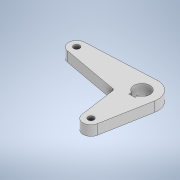
# Autodesk Inventor part: Part3
Saved by Autodesk Inventor 2021 (Build 250183000, 183)
## iProperties
Created: 2022-04-24
Part Number: Part3
Material: Generic
Document SubType Name: Modeling
Designer: hp
Density: 1 g/cm^3
Appearance: Default
Author: hp
Autodesk Inventor part; units mm, degrees
ref_plane "YZ Plane" through (0, 0, 0) normal (1, 0, 0) x (0, 1, 0)
ref_plane "XZ Plane" through (0, 0, 0) normal (0, 1, 0) x (-1, 0, 0)
ref_plane "XY Plane" through (0, 0, 0) normal (0, 0, 1) x (1, 0, 0)
sketch "Sketch1" plane through (0, 0, 0) normal (0, 1, 0) x (-1, 0, 0)
  arc A0 (32.9765, -145.5888) -> (49.4852, -164.4428) centre (48.7166, -148.4613) ccw
  arc A1 (119.1009, -161.0946) -> (120.1528, -145.2338) centre (118.7166, -153.1038) ccw
  arc A2 (57.63, -97.3385) -> (41.8392, -97.025) centre (49.7092, -98.4613) ccw
  line L0 (41.8392, -97.025) -> (32.9765, -145.5888)
  line L1 (49.4852, -164.4428) -> (119.1009, -161.0946)
  line L2 (120.1528, -145.2338) -> (64.3577, -135.0515)
  line L3 (57.63, -97.3385) -> (62.7366, -133.3646)
  circle A3 centre (49.7092, -98.4613) radius 3
  arc A4 (45.7166, -141.0451) -> (51.7166, -141.0451) centre (48.7166, -148.4613) ccw
  circle A5 centre (118.7166, -153.1038) radius 3
  line L4 (51.7166, -138.4613) -> (45.7166, -138.4613)
  line L5 (51.7166, -156.4613) -> (51.7166, -155.8775)
  line L6 (51.7166, -141.0451) -> (51.7166, -138.4613)
  line L7 (45.7166, -138.4613) -> (45.7166, -141.0451)
  arc A6 (62.7366, -133.3646) -> (64.3577, -135.0515) centre (64.7168, -133.0839) ccw
  point P0 (0, 0)
  dimension "d0" = 70
  dimension "d1" = 50
  dimension "d2" = 8
  dimension "d3" = 6
  dimension "d4" = 6
  dimension "d5" = 8
  dimension "d6" = 16
  dimension "d7" = 16
  dimension "d8" = 18
  dimension "d9" = 6
  dimension "d12" = 2
  constraints: 16 end point, 11 point on circle, 10 tangent, 7 centre point, 3 coincident, 2 parallel, 2 perpendicular, 1 horizontal
  measures "d0" horizontal distance of A1.centre A0.centre
  measures "d1" vertical distance of A2.centre A0.centre
  measures "d2" radius of A1
  measures "d3" diameter of A5
  measures "d4" diameter of A3
  measures "d5" radius of A2
  measures "d6" radius of A0
  measures "d7" diameter of A4
  measures "d8" distance of L5.start L4.start
  measures "d9" distance of L4.start L4.end
  measures "d12" radius of A6
extrude "Extrusion1" add sketch "Sketch1" along normal blind 10
equation "\"d10\" = 0.5 * d9"
body "Solid1"
